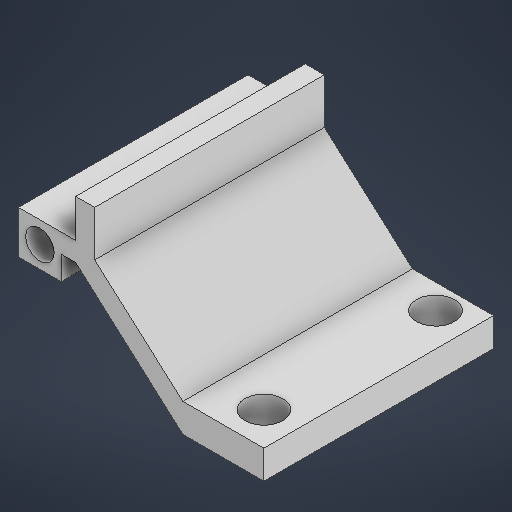
# Autodesk Inventor part: suport3_pcb_temp
Saved by Autodesk Inventor 2026.1 (Build 301233000, 233)
## iProperties
Created: 2025-09-26
Part Number: suport3_pcb_temp
Material: Generic
Document SubType Name: Modeling
Designer: emanuel
Density: 1 g/cm^3
Appearance: Default
Author: emanuel
Autodesk Inventor part; units mm, degrees
ref_plane "YZ Plane" through (0, 0, 0) normal (1, 0, 0) x (0, 1, 0)
ref_plane "XZ Plane" through (0, 0, 0) normal (0, 1, 0) x (-1, 0, 0)
ref_plane "XY Plane" through (0, 0, 0) normal (0, 0, 1) x (1, 0, 0)
sketch "Sketch1" plane through (0, 0, 0) normal (0, 1, 0) x (-1, 0, 0)
  line L0 (0, 0) -> (0, -18)
  circle A0 centre (0, 0) radius 2
  circle A1 centre (0, -18) radius 2
  line L1 (0, -18) -> (5, -18)
  line L2 (5, -18) -> (5, -20.5922)
  line L3 (5, -20.5922) -> (0, -20.5922)
  line L4 (0, -20.5922) -> (0, -18)
  line L5 (0, 0) -> (-3.5, 0)
  line L6 (-3.5, 0) -> (-3.5, 3.5)
  line L7 (-3.5, 3.5) -> (0, 3.5)
  line L8 (0, 3.5) -> (0, 0)
  line L9 (-3.5, 3.5) -> (5, 3.5)
  line L10 (5, 3.5) -> (5, -20.5922)
  line L11 (5, -20.5922) -> (-3.5, -20.5922)
  line L12 (-3.5, -20.5922) -> (-3.5, 3.5)
  dimension "d0" = 18
  dimension "d1" = 4
  dimension "d2" = 4
  dimension "d3" = 5
  dimension "d4" = 3.5
  dimension "d5" = 3.5
  constraints: 26 end point, 6 parallel, 3 horizontal, 3 perpendicular, 2 centre point, 2 coincident, 1 vertical
  measures "d0" distance of L0.start L0.end
  measures "d1" diameter of A0
  measures "d2" diameter of A1
  measures "d3" distance of L2.end L3.end
  measures "d4" distance of L6.end L7.end
  measures "d5" distance of L5.end L6.end
extrude "Extrusion1" add sketch "Sketch1" along normal blind 3 contours A0 L8 L9 L10 L1 A1 L0 | L0 A1 L4 L11 L12 L5 A0 | L5 L6 L7 L8 A0 | L1 L2 L3 L4 A1
sketch "Sketch2" plane through (-5, 0, 3.5) normal (0, 0, 1) x (1, 0, 0)
  line L0 (0, 3) -> (4.25, 3)
  line L1 (0, 3) -> (8.5, 3) projected
  line L2 (4.25, 3) -> (-96.75, 3)
  line L3 (-46.25, 3) -> (-11.25, 3)
  line L4 (-11.25, 3) -> (-11.25, 13)
  line L5 (-11.25, 13) -> (0, 3)
  line L6 (-11.25, 13) -> (-11.25, 10)
  line L7 (0, 0) -> (0, 3) projected
  line L8 (-11.25, 10) -> (0, 0)
  line L9 (-11.25, 10) -> (-17.25, 10)
  line L10 (-17.25, 10) -> (-17.25, 12)
  line L11 (-17.25, 12) -> (-11.25, 12)
  line L12 (-11.25, 12) -> (-11.25, 10)
  line L13 (-11.25, 10) -> (-9.25, 10)
  line L14 (-9.25, 10) -> (-9.25, 16)
  line L15 (-9.25, 16) -> (-11.25, 16)
  line L16 (-11.25, 16) -> (-11.25, 10)
  line L17 (-17.25, 10) -> (-12.75, 10)
  line L18 (-12.75, 10) -> (-12.75, 7.5)
  line L19 (-12.75, 7.5) -> (-17.25, 7.5)
  line L20 (-17.25, 7.5) -> (-17.25, 10)
  line L21 (-15, 10) -> (-15, 9.75)
  circle A0 centre (-15, 9.75) radius 1.5
  point P0 (5, 0)
  point P1 (-11.25, 12)
  point P2 (-11.25, 13)
  point P3 (-9.25, 11.2222)
  dimension "d8" = 101
  dimension "d9" = 35
  dimension "d10" = 10
  dimension "d11" = 3
  dimension "d12" = 6
  dimension "d13" = 2
  dimension "d17" = 2
  dimension "d18" = 6
  dimension "d25" = 4.5
  dimension "d26" = 2.5
  dimension "d27" = 0.25
  dimension "d28" = 3
  constraints: 40 end point, 6 parallel, 4 horizontal, 4 perpendicular, 3 midpoint, 2 point on line, 1 centre point, 1 coincident, 1 vertical
  measures "d8" distance of L0.end L2.end
  measures "d9" distance of L3.start L3.end
  measures "d10" distance of L3.end L4.end
  measures "d11" distance of L4.end L6.end
  measures "d12" distance of L10.end L11.end
  measures "d13" distance of L9.end L10.end
  measures "d17" distance of L15.end L14.end
  measures "d18" distance of L14.end L13.end
  measures "d25" distance of L18.end L19.end
  measures "d26" distance of L17.end L18.end
  measures "d27" distance of L21.start L21.end
  measures "d28" diameter of A0
extrude "Extrusion2" add sketch "Sketch2" against normal up to surface (24.0922 mm away) contours L7 L8 L2 | L2 L8 L13 L14 L5 | L14 L13 L4 L5 | L5 L16 L15 L14 | L9 A0 L10 L11 L4 | L18 L19 L20 L9 A0
body "Solid1"
